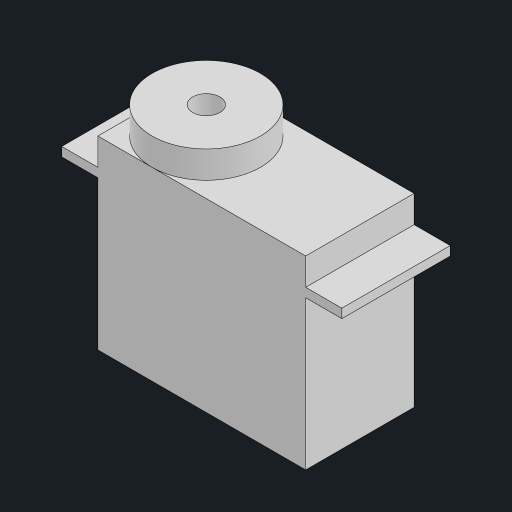
# Autodesk Inventor part: ServoMotor_8g
Saved by Autodesk Inventor 2023 (Build 270158000, 158)
## iProperties
Created: 2022-06-06
Part Number: ServoMotor_8g
Material: Generic
Document SubType Name: Modeling
Designer: legot
Density: 1 g/cm^3
Appearance: Default
Author: legot
Autodesk Inventor part; units mm, degrees
ref_plane "YZ Plane" through (0, 0, 0) normal (1, 0, 0) x (0, 1, 0)
ref_plane "XZ Plane" through (0, 0, 0) normal (0, 1, 0) x (-1, 0, 0)
ref_plane "XY Plane" through (0, 0, 0) normal (0, 0, 1) x (1, 0, 0)
sketch "スケッチ1" plane through (0, 0, 0) normal (0, 1, 0) x (-1, 0, 0)
  line L0 (0, 0) -> (-23, 0)
  line L1 (-23, 0) -> (-23, -12)
  line L2 (-23, -12) -> (0, -12)
  line L3 (0, -12) -> (0, 0)
  dimension "d0" = 23
  dimension "d1" = 12
  constraints: 8 end point, 2 parallel, 1 horizontal, 1 perpendicular
  measures "d0" distance of L1.end L2.end
  measures "d1" distance of L0.end L1.end
extrude "押し出し1" add sketch "スケッチ1" along normal blind 16.5
sketch "スケッチ2" plane through (0, 16.5, 0) normal (0, 1, 0) x (1, 0, 0)
  line L0 (23, 0) -> (23, 12) projected
  line L1 (23, 12) -> (0, 12) projected
  line L2 (0, 12) -> (0, 0) projected
  line L3 (0, 0) -> (23, 0) projected
  line L4 (-4, 0) -> (27, 0)
  line L5 (27, 0) -> (27, 12)
  line L6 (27, 12) -> (-4, 12)
  line L7 (-4, 12) -> (-4, 0)
  dimension "d4" = 4
  dimension "d5" = 4
  constraints: 8 end point, 2 collinear, 2 parallel, 1 horizontal, 1 perpendicular
  measures "d4" distance between parallel lines of L7 L2
  measures "d5" distance between parallel lines of L0 L5
extrude "押し出し2" add sketch "スケッチ2" along normal blind 1
sketch "スケッチ3" plane through (0, 17.5, 0) normal (0, 1, 0) x (1, 0, 0)
  line L0 (-4, 0) -> (27, 0) projected
  line L1 (27, 12) -> (-4, 12) projected
  line L2 (0, 12) -> (0, 0) projected
  line L3 (23, 0) -> (23, 12) projected
extrude "押し出し3" add sketch "スケッチ3" along normal blind 3
sketch "スケッチ4" plane through (0, 20.5, 0) normal (0, 1, 0) x (1, 0, 0)
  line L0 (23, 12) -> (0, 12) projected
  line L1 (0, 12) -> (0, 0) projected
  line L2 (0, 0) -> (23, 0) projected
  circle A0 centre (6, 6) radius 6
  constraints: 3 tangent, 1 centre point
extrude "押し出し4" add sketch "スケッチ4" along normal blind 3 contours A0
sketch "スケッチ5" plane through (6, 23.5, -6) normal (0, 1, 0) x (1, 0, 0)
  circle A0 centre (0, 0) radius 6 projected
  point P0 (-6, -6)
  constraints: 1 coincident
hole "穴1" at (6, 23.5, -6) direction (0, -1, 0) diameter 3 end through all
equation "\"d5\" = d4"
